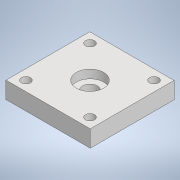
# Autodesk Inventor part: Shoulderbottom
Saved by Autodesk Inventor 2022 (Build 260153000, 153)
## iProperties
Created: 2022-03-24
Part Number: Shoulderbottom
Material: Genérico
Document SubType Name: Modeling
Designer: JK
Density: 1 g/cm^3
Appearance: Valor por defecto
Author: JK
Autodesk Inventor part; units mm, degrees
ref_plane "YZ Plane" through (0, 0, 0) normal (1, 0, 0) x (0, 1, 0)
ref_plane "XZ Plane" through (0, 0, 0) normal (0, 1, 0) x (-1, 0, 0)
ref_plane "XY Plane" through (0, 0, 0) normal (0, 0, 1) x (1, 0, 0)
sketch "Boceto1" plane through (0, 0, 0) normal (0, 1, 0) x (-1, 0, 0)
  line L0 (-25, 24.85) -> (25, 24.85)
  line L1 (25, 24.85) -> (25, -24.85)
  line L2 (25, -24.85) -> (-25, -24.85)
  line L3 (-25, -24.85) -> (-25, 24.85)
  line L4 (-25, 24.85) -> (25, -24.85) construction
  line L5 (25, 24.85) -> (-25, -24.85) construction
  circle A0 centre (0, 0) radius 4.35
  dimension "d0" = 50
  dimension "d1" = 8.7
  dimension "d2" = 49.7
  constraints: 12 end point, 2 midpoint, 2 parallel, 1 centre point, 1 coincident, 1 horizontal, 1 perpendicular
  measures "d0" distance of L0.start L0.end
  measures "d1" diameter of A0
  measures "d2" distance of L0.end L1.end
extrude "Extrusión1" add sketch "Boceto1" along normal blind 10
sketch "Boceto4" plane through (0, 0, 0) normal (0, -1, 0) x (1, 0, 0)
  line L0 (25, 24.85) -> (25, -24.85) projected
  line L1 (-25, -24.85) -> (-25, 24.85) projected
  line L2 (25, 24.85) -> (-25, 24.85)
  line L3 (-25, 24.85) -> (-25, 17.85)
  line L4 (-25, 17.85) -> (25, 17.85)
  line L5 (25, 17.85) -> (25, 24.85)
  line L6 (25, -24.85) -> (-25, -24.85) projected
  line L7 (25, -24.85) -> (-25, -24.85)
  line L8 (-25, -24.85) -> (-25, -17.85)
  line L9 (-25, -17.85) -> (25, -17.85)
  line L10 (25, -17.85) -> (25, -24.85)
  line L11 (25, -24.85) -> (-25, -24.85) projected
  line L12 (25, 24.85) -> (25, -24.85) projected
  line L13 (-25, 24.85) -> (25, 24.85) projected
  line L14 (-25, -24.85) -> (-25, 24.85) projected
  circle A0 centre (0, 0) radius 4.35 projected
  point P0 (-25, -17.85)
  point P1 (25, -17.85)
  point P2 (-25, 24.85)
  dimension "d14" = 7
  dimension "d15" = 7
  constraints: 16 end point, 4 parallel, 2 horizontal, 2 perpendicular, 2 point on line
  measures "d14" distance between parallel lines of L4 L2
  measures "d15" distance between parallel lines of L6 L9
extrude "Extrusión4" [suppressed]
sketch "Boceto5" plane through (0, 0, 0) normal (0, 0, 1) x (1, 0, 0)
  circle A0 centre (18, -5.5) radius 2.7
  circle A1 centre (-18, -5.5) radius 2.7
  line L0 (20, -12) -> (-20, -12) projected
  line L1 (25, 0) -> (25, 10) projected
  line L2 (-25, 0) -> (-25, 10) projected
  point P0 (0, 0)
  point P1 (-25, 10)
  dimension "d19" = 6.5
  dimension "d20" = 5.4
  dimension "d21" = 7
  dimension "d22" = 7
  constraints: 2 centre point, 1 equal radius, 1 horizontal alignment, 2 other
  measures "d19" distance from line of L0 A0.centre
  measures "d20" diameter of A0
extrude "Extrusión5" [suppressed]
sketch "Boceto6" plane through (0, 0, 0) normal (0, 0, 1) x (1, 0, 0)
  circle A0 centre (13, -5.5) radius 2.7 projected
  circle A1 centre (13, -5.5) radius 4.65
  circle A2 centre (-13, -5.5) radius 2.7 projected
  circle A3 centre (-13, -5.5) radius 4.65
  point P0 (0, 0)
  dimension "d25" = 9.3
  constraints: 2 centre point, 2 coincident, 1 equal radius
  measures "d25" diameter of A1
extrude "Extrusión6" [suppressed]
fillet "Empalme2" [suppressed]
fillet "Empalme3" [suppressed]
sketch "Boceto8" plane through (0, 0, 0) normal (0, -1, 0) x (1, 0, 0)
  circle A0 centre (0, 0) radius 4.35 projected
  line L0 (-25, -24.85) -> (-25, 24.85) projected
  line L1 (25, 24.85) -> (25, -24.85) projected
  circle A1 centre (0, 0) radius 7.5
  line L2 (25, -24.85) -> (-25, -24.85) projected
  line L3 (-25, 24.85) -> (25, 24.85) projected
  dimension "d30" = 15
  constraints: 1 centre point, 1 coincident
  measures "d30" diameter of A1
extrude "Extrusión7" [suppressed]
fillet "Empalme4" [suppressed]
sketch "Boceto9" plane through (0, 10, 0) normal (0, 1, 0) x (1, 0, 0)
  circle A0 centre (0, 0) radius 8.125
  dimension "d34" = 16.25
  constraints: 1 centre point, 1 coincident
  measures "d34" diameter of A0
extrude "Extrusión8" cut sketch "Boceto9" against normal blind 5
sketch "Boceto10" plane through (0, 0, 0) normal (0, -1, 0) x (1, 0, 0)
  circle A0 centre (-18.9971, -19.0029) radius 2.7 projected
  circle A1 centre (-19.0029, 18.9971) radius 2.7 projected
  circle A2 centre (19.0029, -18.9971) radius 2.7 projected
  circle A3 centre (18.9971, 19.0029) radius 2.7 projected
  point P0 (0, 0)
extrude "Extrusión9" cut sketch "Boceto10" against normal through all
fillet "Empalme5" radius 5 4 edges at (-25, 5, 24.85) (25, 5, 24.85) (25, 5, -24.85) (-25, 5, -24.85)
sketch "Boceto11" plane through (0, 0, 0) normal (0, -1, 0) x (1, 0, 0)
  circle A0 centre (19.0029, -18.9971) radius 2.7 projected
  circle A1 centre (19.0029, -18.9971) radius 4.05
  line L0 (14.9529, -21.3354) -> (14.9529, -16.6588)
  line L1 (14.9529, -16.6588) -> (19.0029, -14.3206)
  line L2 (19.0029, -14.3206) -> (23.0529, -16.6588)
  line L3 (23.0529, -16.6588) -> (23.0529, -21.3354)
  line L4 (23.0529, -21.3354) -> (19.0029, -23.6737)
  line L5 (19.0029, -23.6737) -> (14.9529, -21.3354)
  point P0 (0, 0)
  dimension "d40" = 8.1
  constraints: 12 end point, 2 coincident, 1 centre point, 1 tangent, 1 vertical, 13 other
  measures "d40" diameter of A1
extrude "Extrusión10" cut sketch "Boceto11" against normal blind 4 contours A0 | A1 | L3 L4 A1 | A1 L2 L3 | A1 L1 L2 | L4 L5 A1 | A1 L0 L1 | L5 L0 A1
pattern_circular "Patrón circular1" count 4 over 360 about axis through (0, 0, 0) along (0, 1, 0) of "Extrusión10"
